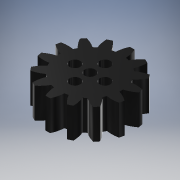
# Autodesk Inventor part: Spur Gear1
Saved by Autodesk Inventor 2017 SP1 (Build 210196100, 196)
## iProperties
Created: 2019-09-22
Part Number: Spur Gear1
Material: ABS Plastic
Document SubType Name: Modeling
Designer: Zach
Categories: <?xml version="1.0" encoding="UTF-16"?> <MemberInstance><Categories><FamilyTemplate><FamilyTemplateParameter ValueType="xs:double" Id="1" ObjectReferenceKey="da_z" ObjectType="kUserParameterObject"/><FamilyTemplateParameter ValueType="xs:double" Id="2" ObjectReferenceKey="da_b" ObjectType="kUserParameterObject"/><FamilyTemplateParameter ValueType="xs:double" Id="3" ObjectReferenceKey="da_beta" ObjectType="kUserParameterObject"/><FamilyTemplateParameter ValueType="xs:double" Id="4" ObjectReferenceKey="da_da" ObjectType="kUserParameterObject"/><FamilyTemplateParameter ValueType="xs:double" Id="5" ObjectReferenceKey="da_aw" ObjectType="kUserParameterObject"/><FamilyTemplateParameter ValueType="xs:string" Id="6" ObjectReferenceKey="EAIAABAAAACIAQAAAAAAAIAAAAAAAAAA" ObjectType="83910656" SubObjectId="SurfaceGeometry"/></FamilyTemplate><ParamToTemplateMap><ParamToTemplate CategoryParameter="//CategoryParameter[@InternalName='046C89C9-8512-4d59-83FE-43B91F4F132A']" TemplateParameter="1"/><ParamToTemplate CategoryParameter="//CategoryParameter[@InternalName='2552DF32-E462-4b46-AEBF-C6C7768E72AC']" TemplateParameter="2"/><ParamToTemplate CategoryParameter="//CategoryParameter[@InternalName='C9EE641D-15FC-4fae-A226-E94C4372FDD7']" TemplateParameter="3"/><ParamToTemplate><ParamToTemplate CategoryParameter="//CategoryParameter[@InternalName='00B6519A-459B-49c7-AD84-2E56D39A5744']" ConstantValue="0.000000"/></ParamToTemplate><ParamToTemplate><ParamToTemplate CategoryParameter="//CategoryParameter[@InternalName='04B31F0E-C7A6-4894-AA32-9629BEFACF47']" ConstantValue="1.000000"/></ParamToTemplate><ParamToTemplate><ParamToTemplate CategoryParameter="//CategoryParameter[@InternalName='43CBEC2E-7847-49e7-A936-2F7889FCB2D9']" ConstantValue="0.250000"/></ParamToTemplate><ParamToTemplate><ParamToTemplate CategoryParameter="//CategoryParameter[@InternalName='B1EFC894-105D-4ebd-86BF-FA20ED196853']" ConstantValue="0.350000"/></ParamToTemplate><ParamToTemplate><ParamToTemplate CategoryParameter="//CategoryParameter[@InternalName='51175063-3D10-4879-93E8-6246FE8B403D']" ConstantValue="2060000000.000000"/></ParamToTemplate><ParamToTemplate><ParamToTemplate CategoryParameter="//CategoryParameter[@InternalName='A3A52E27-4454-46a9-B0BD-C932399B70AF']" ConstantValue="0.300000"/></ParamToTemplate><ParamToTemplate><ParamToTemplate CategoryParameter="//CategoryParameter[@InternalName='91B76062-C214-41d9-B1B9-14D2AB99603D']" ConstantValue="0.180000"/></ParamToTemplate><ParamToTemplate><ParamToTemplate CategoryParameter="//CategoryParameter[@InternalName='374E806E-8B8A-4dda-A9AA-1039D6500AD2']" ConstantValue="5.555556"/></ParamToTemplate><ParamToTemplate><ParamToTemplate CategoryParameter="//CategoryParameter[@InternalName='2D373A89-B862-43d6-8D0B-0CBF12AB9F6C']" ConstantValue="0.392699"/></ParamToTemplate><ParamToTemplate CategoryParameter="//CategoryParameter[@InternalName='37777632-D6A2-4fac-9D53-DB8ACD95C989']" TemplateParameter="4"/><ParamToTemplate CategoryParameter="//CategoryParameter[@InternalName='FD1017F1-B727-4f7e-9707-0F86F1FF9423']" TemplateParameter="5"/><ParamToTemplate><ParamToTemplate CategoryParameter="//CategoryParameter[@InternalName='9E1B4470-B2D3-4ff1-B813-535BB4CDF51A']" ConstantValue="3520000.000000"/></ParamToTemplate><ParamToTemplate><ParamToTemplate CategoryParameter="//CategoryParameter[@InternalName='F8452263-BFF6-458c-9FB1-07C4B99E95CD']" ConstantValue="11400000.000000"/></ParamToTemplate><ParamToTemplate><ParamToTemplate CategoryParameter="//CategoryParameter[@InternalName='3E3BB259-FD49-497f-8171-6EBC954A3479']" ConstantValue="2.000000"/></ParamToTemplate><ParamToTemplate CategoryParameter="//CategoryParameter[@InternalName='27C3BAF2-7550-4e4b-AE2C-0DB134B7D9B7']" TemplateParameter="6"/></ParamToTemplateMap><Category DisplayName="Gear" InternalName="DC85795E-93AB-48d5-8EEE-5A27447B64BD" Mnemonic="Gear"><CategoryParameter DisplayName="z" InternalName="046C89C9-8512-4d59-83FE-43B91F4F132A" Mnemonic="z"/><CategoryParameter DisplayName="b" InternalName="2552DF32-E462-4b46-AEBF-C6C7768E72AC" Mnemonic="b"/><CategoryParameter DisplayName="||b|" InternalName="C9EE641D-15FC-4fae-A226-E94C4372FDD7" Mnemonic="beta"/><CategoryParameter DisplayName="x" InternalName="00B6519A-459B-49c7-AD84-2E56D39A5744" Mnemonic="x"/><CategoryParameter DisplayName="a*" InternalName="04B31F0E-C7A6-4894-AA32-9629BEFACF47" Mnemonic="a"/><CategoryParameter DisplayName="c*" InternalName="43CBEC2E-7847-49e7-A936-2F7889FCB2D9" Mnemonic="c"/><CategoryParameter DisplayName="r|.f|*" InternalName="B1EFC894-105D-4ebd-86BF-FA20ED196853" Mnemonic="rf"/><CategoryParameter DisplayName="E" InternalName="51175063-3D10-4879-93E8-6246FE8B403D" Mnemonic="E"/><CategoryParameter DisplayName="||m|" InternalName="A3A52E27-4454-46a9-B0BD-C932399B70AF" Mnemonic="mi"/><Category DisplayName="SpurGear" InternalName="26C5A22E-A91E-4dfd-A3B3-23CCAFAE1764" Mnemonic="SpurGear"><CategoryParameter DisplayName="m" InternalName="91B76062-C214-41d9-B1B9-14D2AB99603D" Mnemonic="m"/><CategoryParameter DisplayName="P" InternalName="374E806E-8B8A-4dda-A9AA-1039D6500AD2" Mnemonic="PP"/><CategoryParameter DisplayName="||a|" InternalName="2D373A89-B862-43d6-8D0B-0CBF12AB9F6C" Mnemonic="alpha"/><CategoryParameter DisplayName="d|.a|" InternalName="37777632-D6A2-4fac-9D53-DB8ACD95C989" Mnemonic="da"/><CategoryParameter DisplayName="a|.w|" InternalName="FD1017F1-B727-4f7e-9707-0F86F1FF9423" Mnemonic="aw"/><CategoryParameter DisplayName="||s||.Flim|" InternalName="9E1B4470-B2D3-4ff1-B813-535BB4CDF51A" Mnemonic="sFlim"/><CategoryParameter DisplayName="||s||.Hlim|" InternalName="F8452263-BFF6-458c-9FB1-07C4B99E95CD" Mnemonic="sHlim"/><CategoryParameter DisplayName="type" InternalName="3E3BB259-FD49-497f-8171-6EBC954A3479" Mnemonic="type"/><CategoryParameter DisplayName="PitchDiameter" InternalName="27C3BAF2-7550-4e4b-AE2C-0DB134B7D9B7" Mnemonic="IDS_PITCHDIAM"/></Category></Category></Categories></MemberInstance>
Density: 1.06 g/cm^3
Appearance: Smooth - Black
CustomPartVersion: 1
Author: Zach
Autodesk Inventor part; units mm, degrees
ref_plane "YZ Plane" through (0, 0, 0) normal (1, 0, 0) x (0, 1, 0)
ref_plane "XZ Plane" through (0, 0, 0) normal (0, 1, 0) x (-1, 0, 0)
ref_plane "XY Plane" through (0, 0, 0) normal (0, 0, 1) x (1, 0, 0)
sketch "Sketch1" plane through (0, 0, 0) normal (0, 0, 1) x (1, 0, 0)
  circle A0 centre (0, 0) radius 14
  dimension "d0" = 28
  constraints: 1 centre point
  measures "d0" diameter of A0
extrude "Extrusion1" add sketch "Sketch1" along normal blind 10
ref_plane "Work Plane2" through (0, 0, 5) normal (0, 0, 1) x (1, 0, 0)
sketch "Sketch2" plane through (0, 0, 0) normal (0, 0, -1) x (-1, 0, 0)
  circle A0 centre (0, 0) radius 14 projected
  circle A1 centre (0, 0) radius 12.7647
  dimension "d3" = 25.5294
  constraints: 1 centre point, 1 coincident
  measures "d3" diameter of A1
surface extrude "Pitch Diameter" sketch "Sketch2" against normal through all shown no curves A1
ref_plane "Work Plane8" through (0, 0, 0) normal (0.9749279, 0.2225209, 0) x (0, 0, 1)
ref_plane "Work Plane9" through (0, 0, 0) normal (1, 0, 0) x (0, 1, 0)
spur gear teeth "Spur Gear" teeth 14 pitch diameter 25.2 tip diameter 28 root diameter 20.7 face width 10 start plane through (0, 0, 0) normal (0, 0, -1) x (-1, 0, 0)
sketch "Sketch4" plane through (0, 0, 10) normal (0, 0, 1) x (1, 0, 0)
  circle A0 centre (0, 0) radius 16
  circle A1 centre (12, 0) radius 2.5
  circle A2 centre (12, 0) radius 4.5
  circle A3 centre (0, 0) radius 7.5
  dimension "d49" = 32
  dimension "d50" = 5
  dimension "d51" = 12
  dimension "d52" = 9
  constraints: 4 centre point, 3 coincident, 1 horizontal alignment, 1 tangent
  measures "d49" diameter of A0
  measures "d50" diameter of A1
  measures "d51" distance of point (0, 0) A1.centre
  measures "d52" diameter of A2
extrude "Extrusion2" [suppressed]
sketch "Sketch5" plane through (0, 0, 16) normal (0, 0, 1) x (1, 0, 0)
  circle A0 centre (0, 0) radius 16
  circle A1 centre (12, 0) radius 2.5
  circle A2 centre (0, 12) radius 2.5
  circle A3 centre (-12, 0) radius 2.5
  circle A4 centre (0, -12) radius 2.5
  dimension "d55" = 32
  dimension "d56" = 5
  dimension "d57" = 12
  dimension "d60" = 360
  constraints: 5 centre point, 1 coincident, 1 horizontal alignment, 9 other
  measures "d55" diameter of A0
  measures "d56" diameter of A1
  measures "d57" distance of A1.centre point (0, 0)
extrude "Extrusion3" [suppressed]
sketch "Sketch6" plane through (0, 0, 18) normal (0, 0, 1) x (1, 0, 0)
  circle A0 centre (0, -12) radius 2.5 projected
  line L0 (2.5, -12) -> (2.5, -16)
  line L1 (2.5, -16) -> (-2.5, -16)
  line L2 (-2.5, -16) -> (-2.5, -12)
  circle A1 centre (0, 0) radius 16 construction
  arc A2 (2.5, -12) -> (-2.5, -12) centre (0, -12) ccw
  line L3 (12, 2.5) -> (16, 2.5)
  line L4 (16, 2.5) -> (16, -2.5)
  line L5 (16, -2.5) -> (12, -2.5)
  arc A3 (12, 2.5) -> (12, -2.5) centre (12, 0) ccw
  line L6 (-2.5, 12) -> (-2.5, 16)
  line L7 (-2.5, 16) -> (2.5, 16)
  line L8 (2.5, 16) -> (2.5, 12)
  arc A4 (-2.5, 12) -> (2.5, 12) centre (0, 12) ccw
  line L9 (-12, -2.5) -> (-16, -2.5)
  line L10 (-16, -2.5) -> (-16, 2.5)
  line L11 (-16, 2.5) -> (-12, 2.5)
  arc A5 (-12, -2.5) -> (-12, 2.5) centre (-12, 0) ccw
  point P0 (12, 0)
  point P1 (0, 12)
  point P2 (-12, 0)
  dimension "d66" = 360
  constraints: 24 end point, 10 point on circle, 5 tangent, 4 centre point, 1 horizontal alignment, 1 perpendicular, 1 vertical, 41 other
extrude "Extrusion4" [suppressed]
sketch "Sketch7" plane through (0, 0, 13) normal (0, 0, -1) x (-1, 0, 0)
  arc A0 (6.7721, 12.2531) -> (5.3576, 12.9343) centre (0, 0) ccw projected
  arc A1 (-2.5, 12) -> (2.5, 12) centre (0, 12) ccw projected
  arc A2 (-12, -2.5) -> (-12, 2.5) centre (-12, 0) ccw projected
  arc A3 (2.5, -12) -> (-2.5, -12) centre (0, -12) ccw projected
  arc A4 (12, 2.5) -> (12, -2.5) centre (12, 0) ccw projected
  circle A5 centre (0, 12) radius 4.5
  circle A6 centre (-12, 0) radius 4.5
  circle A7 centre (0, -12) radius 4.5
  circle A8 centre (12, 0) radius 4.5
  arc A9 (0.785, 13.978) -> (-0.785, 13.978) centre (0, 0) ccw projected
  arc A10 (5.9892, 8.4411) -> (6.7721, 12.2531) centre (-4.1276, 12.505) ccw projected
  arc A11 (5.3576, 12.9343) -> (2.8652, 9.9455) centre (12.3503, 4.5696) ccw projected
  arc A12 (2.8652, 9.9455) -> (1.7337, 10.2038) centre (0, 0) ccw projected
  arc A13 (1.7337, 10.2038) -> (0.785, 13.978) centre (-9.1446, 9.4757) ccw projected
  arc A14 (-0.785, 13.978) -> (-1.7337, 10.2038) centre (9.1446, 9.4757) ccw projected
  arc A15 (-1.7337, 10.2038) -> (-2.8652, 9.9455) centre (0, 0) ccw projected
  arc A16 (-2.8652, 9.9455) -> (-5.3576, 12.9343) centre (-12.3503, 4.5696) ccw projected
  arc A17 (-5.3576, 12.9343) -> (-6.7721, 12.2531) centre (0, 0) ccw projected
  arc A18 (-6.7721, 12.2531) -> (-5.9892, 8.4411) centre (4.1276, 12.505) ccw projected
  arc A19 (-5.9892, 8.4411) -> (-6.8967, 7.7174) centre (0, 0) ccw projected
  arc A20 (-6.8967, 7.7174) -> (-10.439, 9.3289) centre (-13.11, -1.2415) ccw projected
  arc A21 (-10.439, 9.3289) -> (-11.4179, 8.1014) centre (0, 0) ccw projected
  arc A22 (-11.4179, 8.1014) -> (-9.0586, 5.0065) centre (-1.7068, 13.0575) ccw projected
  arc A23 (-9.0586, 5.0065) -> (-9.5622, 3.9608) centre (0, 0) ccw projected
  arc A24 (-9.5622, 3.9608) -> (-13.4528, 3.8757) centre (-11.273, -6.8068) ccw projected
  arc A25 (-13.4528, 3.8757) -> (-13.8022, 2.3451) centre (0, 0) ccw projected
  arc A26 (-13.8022, 2.3451) -> (-10.3337, 0.5803) centre (-7.2032, 11.0239) ccw projected
  arc A27 (-10.3337, 0.5803) -> (-10.3337, -0.5803) centre (0, 0) ccw projected
  arc A28 (-10.3337, -0.5803) -> (-13.8022, -2.3451) centre (-7.2032, -11.0239) ccw projected
  arc A29 (-13.8022, -2.3451) -> (-13.4528, -3.8757) centre (0, 0) ccw projected
  arc A30 (-13.4528, -3.8757) -> (-9.5622, -3.9608) centre (-11.273, 6.8068) ccw projected
  arc A31 (-9.5622, -3.9608) -> (-9.0586, -5.0065) centre (0, 0) ccw projected
  arc A32 (-9.0586, -5.0065) -> (-11.4179, -8.1014) centre (-1.7068, -13.0575) ccw projected
  arc A33 (-11.4179, -8.1014) -> (-10.439, -9.3289) centre (0, 0) ccw projected
  arc A34 (-10.439, -9.3289) -> (-6.8967, -7.7174) centre (-13.11, 1.2415) ccw projected
  arc A35 (-6.8967, -7.7174) -> (-5.9892, -8.4411) centre (0, 0) ccw projected
  arc A36 (-5.9892, -8.4411) -> (-6.7721, -12.2531) centre (4.1276, -12.505) ccw projected
  arc A37 (-6.7721, -12.2531) -> (-5.3576, -12.9343) centre (0, 0) ccw projected
  arc A38 (-5.3576, -12.9343) -> (-2.8652, -9.9455) centre (-12.3503, -4.5696) ccw projected
  arc A39 (-2.8652, -9.9455) -> (-1.7337, -10.2038) centre (0, 0) ccw projected
  arc A40 (-1.7337, -10.2038) -> (-0.785, -13.978) centre (9.1446, -9.4757) ccw projected
  arc A41 (-0.785, -13.978) -> (0.785, -13.978) centre (0, 0) ccw projected
  arc A42 (0.785, -13.978) -> (1.7337, -10.2038) centre (-9.1446, -9.4757) ccw projected
  arc A43 (1.7337, -10.2038) -> (2.8652, -9.9455) centre (0, 0) ccw projected
  arc A44 (2.8652, -9.9455) -> (5.3576, -12.9343) centre (12.3503, -4.5696) ccw projected
  arc A45 (5.3576, -12.9343) -> (6.7721, -12.2531) centre (0, 0) ccw projected
  arc A46 (6.7721, -12.2531) -> (5.9892, -8.4411) centre (-4.1276, -12.505) ccw projected
  arc A47 (5.9892, -8.4411) -> (6.8967, -7.7174) centre (0, 0) ccw projected
  arc A48 (6.8967, -7.7174) -> (10.439, -9.3289) centre (13.11, 1.2415) ccw projected
  arc A49 (10.439, -9.3289) -> (11.4179, -8.1014) centre (0, 0) ccw projected
  arc A50 (11.4179, -8.1014) -> (9.0586, -5.0065) centre (1.7068, -13.0575) ccw projected
  arc A51 (9.0586, -5.0065) -> (9.5622, -3.9608) centre (0, 0) ccw projected
  arc A52 (9.5622, -3.9608) -> (13.4528, -3.8757) centre (11.273, 6.8068) ccw projected
  arc A53 (13.4528, -3.8757) -> (13.8022, -2.3451) centre (0, 0) ccw projected
  arc A54 (13.8022, -2.3451) -> (10.3337, -0.5803) centre (7.2032, -11.0239) ccw projected
  arc A55 (10.3337, -0.5803) -> (10.3337, 0.5803) centre (0, 0) ccw projected
  arc A56 (10.3337, 0.5803) -> (13.8022, 2.3451) centre (7.2032, 11.0239) ccw projected
  arc A57 (13.8022, 2.3451) -> (13.4528, 3.8757) centre (0, 0) ccw projected
  arc A58 (13.4528, 3.8757) -> (9.5622, 3.9608) centre (11.273, -6.8068) ccw projected
  arc A59 (9.5622, 3.9608) -> (9.0586, 5.0065) centre (0, 0) ccw projected
  arc A60 (9.0586, 5.0065) -> (11.4179, 8.1014) centre (1.7068, 13.0575) ccw projected
  arc A61 (11.4179, 8.1014) -> (10.439, 9.3289) centre (0, 0) ccw projected
  arc A62 (10.439, 9.3289) -> (6.8967, 7.7174) centre (13.11, -1.2415) ccw projected
  arc A63 (6.8967, 7.7174) -> (5.9892, 8.4411) centre (0, 0) ccw projected
  dimension "d76" = 9
  dimension "d77" = 9
  dimension "d78" = 9
  dimension "d79" = 9
  constraints: 4 centre point, 4 coincident
  measures "d76" diameter of A5
  measures "d77" diameter of A6
  measures "d78" diameter of A7
  measures "d79" diameter of A8
extrude "Extrusion6" [suppressed]
sketch "Sketch8" plane through (0, 0, 13) normal (0, 0, -1) x (-1, 0, 0)
  arc A0 (-2.5, 12) -> (2.5, 12) centre (0, 12) ccw projected
  circle A1 centre (0, 12) radius 4.5
  circle A2 centre (-12, 0) radius 4.5
  circle A3 centre (0, -12) radius 4.5
  circle A4 centre (12, 0) radius 4.5
  point P0 (0, 0)
  dimension "d82" = 9
  dimension "d85" = 360
  constraints: 4 centre point, 1 coincident, 9 other
  measures "d82" diameter of A1
extrude "Extrusion7" [suppressed]
sketch "Sketch18" plane through (0, 0, 10) normal (0, 0, 1) x (1, 0, 0)
  circle A0 centre (5, 0) radius 1.1
  circle A1 centre (0, 5) radius 1.1
  circle A2 centre (-5, 0) radius 1.1
  circle A3 centre (0, -5) radius 1.1
  circle A4 centre (5.6569, 5.6569) radius 1.1
  line L0 (0, 0) -> (5.6569, 5.6569) construction
  line L1 (0, 0) -> (5, 0) construction
  circle A5 centre (-5.6569, 5.6569) radius 1.1
  circle A6 centre (-5.6569, -5.6569) radius 1.1
  circle A7 centre (5.6569, -5.6569) radius 1.1
  circle A8 centre (0, 0) radius 1.1
  arc A9 (0.785, 13.978) -> (-0.785, 13.978) centre (0, 0) ccw projected
  arc A10 (-6.7721, 12.2531) -> (-5.9892, 8.4411) centre (4.1276, 12.505) ccw projected
  arc A11 (-5.3576, 12.9343) -> (-6.7721, 12.2531) centre (0, 0) ccw projected
  arc A12 (-2.8652, 9.9455) -> (-5.3576, 12.9343) centre (-12.3503, 4.5696) ccw projected
  arc A13 (-1.7337, 10.2038) -> (-2.8652, 9.9455) centre (0, 0) ccw projected
  arc A14 (-0.785, 13.978) -> (-1.7337, 10.2038) centre (9.1446, 9.4757) ccw projected
  arc A15 (1.7337, 10.2038) -> (0.785, 13.978) centre (-9.1446, 9.4757) ccw projected
  arc A16 (2.8652, 9.9455) -> (1.7337, 10.2038) centre (0, 0) ccw projected
  arc A17 (5.3576, 12.9343) -> (2.8652, 9.9455) centre (12.3503, 4.5696) ccw projected
  arc A18 (6.7721, 12.2531) -> (5.3576, 12.9343) centre (0, 0) ccw projected
  arc A19 (5.9892, 8.4411) -> (6.7721, 12.2531) centre (-4.1276, 12.505) ccw projected
  arc A20 (6.8967, 7.7174) -> (5.9892, 8.4411) centre (0, 0) ccw projected
  arc A21 (10.439, 9.3289) -> (6.8967, 7.7174) centre (13.11, -1.2415) ccw projected
  arc A22 (11.4179, 8.1014) -> (10.439, 9.3289) centre (0, 0) ccw projected
  arc A23 (9.0586, 5.0065) -> (11.4179, 8.1014) centre (1.7068, 13.0575) ccw projected
  arc A24 (9.5622, 3.9608) -> (9.0586, 5.0065) centre (0, 0) ccw projected
  arc A25 (13.4528, 3.8757) -> (9.5622, 3.9608) centre (11.273, -6.8068) ccw projected
  arc A26 (13.8022, 2.3451) -> (13.4528, 3.8757) centre (0, 0) ccw projected
  arc A27 (10.3337, 0.5803) -> (13.8022, 2.3451) centre (7.2032, 11.0239) ccw projected
  arc A28 (10.3337, -0.5803) -> (10.3337, 0.5803) centre (0, 0) ccw projected
  arc A29 (13.8022, -2.3451) -> (10.3337, -0.5803) centre (7.2032, -11.0239) ccw projected
  arc A30 (13.4528, -3.8757) -> (13.8022, -2.3451) centre (0, 0) ccw projected
  arc A31 (9.5622, -3.9608) -> (13.4528, -3.8757) centre (11.273, 6.8068) ccw projected
  arc A32 (9.0586, -5.0065) -> (9.5622, -3.9608) centre (0, 0) ccw projected
  arc A33 (11.4179, -8.1014) -> (9.0586, -5.0065) centre (1.7068, -13.0575) ccw projected
  arc A34 (10.439, -9.3289) -> (11.4179, -8.1014) centre (0, 0) ccw projected
  arc A35 (6.8967, -7.7174) -> (10.439, -9.3289) centre (13.11, 1.2415) ccw projected
  arc A36 (5.9892, -8.4411) -> (6.8967, -7.7174) centre (0, 0) ccw projected
  arc A37 (6.7721, -12.2531) -> (5.9892, -8.4411) centre (-4.1276, -12.505) ccw projected
  arc A38 (5.3576, -12.9343) -> (6.7721, -12.2531) centre (0, 0) ccw projected
  arc A39 (2.8652, -9.9455) -> (5.3576, -12.9343) centre (12.3503, -4.5696) ccw projected
  arc A40 (1.7337, -10.2038) -> (2.8652, -9.9455) centre (0, 0) ccw projected
  arc A41 (0.785, -13.978) -> (1.7337, -10.2038) centre (-9.1446, -9.4757) ccw projected
  arc A42 (-0.785, -13.978) -> (0.785, -13.978) centre (0, 0) ccw projected
  arc A43 (-1.7337, -10.2038) -> (-0.785, -13.978) centre (9.1446, -9.4757) ccw projected
  arc A44 (-2.8652, -9.9455) -> (-1.7337, -10.2038) centre (0, 0) ccw projected
  arc A45 (-5.3576, -12.9343) -> (-2.8652, -9.9455) centre (-12.3503, -4.5696) ccw projected
  arc A46 (-6.7721, -12.2531) -> (-5.3576, -12.9343) centre (0, 0) ccw projected
  arc A47 (-5.9892, -8.4411) -> (-6.7721, -12.2531) centre (4.1276, -12.505) ccw projected
  arc A48 (-6.8967, -7.7174) -> (-5.9892, -8.4411) centre (0, 0) ccw projected
  arc A49 (-10.439, -9.3289) -> (-6.8967, -7.7174) centre (-13.11, 1.2415) ccw projected
  arc A50 (-11.4179, -8.1014) -> (-10.439, -9.3289) centre (0, 0) ccw projected
  arc A51 (-9.0586, -5.0065) -> (-11.4179, -8.1014) centre (-1.7068, -13.0575) ccw projected
  arc A52 (-9.5622, -3.9608) -> (-9.0586, -5.0065) centre (0, 0) ccw projected
  arc A53 (-13.4528, -3.8757) -> (-9.5622, -3.9608) centre (-11.273, 6.8068) ccw projected
  arc A54 (-13.8022, -2.3451) -> (-13.4528, -3.8757) centre (0, 0) ccw projected
  arc A55 (-10.3337, -0.5803) -> (-13.8022, -2.3451) centre (-7.2032, -11.0239) ccw projected
  arc A56 (-10.3337, 0.5803) -> (-10.3337, -0.5803) centre (0, 0) ccw projected
  arc A57 (-13.8022, 2.3451) -> (-10.3337, 0.5803) centre (-7.2032, 11.0239) ccw projected
  arc A58 (-13.4528, 3.8757) -> (-13.8022, 2.3451) centre (0, 0) ccw projected
  arc A59 (-9.5622, 3.9608) -> (-13.4528, 3.8757) centre (-11.273, -6.8068) ccw projected
  arc A60 (-9.0586, 5.0065) -> (-9.5622, 3.9608) centre (0, 0) ccw projected
  arc A61 (-11.4179, 8.1014) -> (-9.0586, 5.0065) centre (-1.7068, 13.0575) ccw projected
  arc A62 (-10.439, 9.3289) -> (-11.4179, 8.1014) centre (0, 0) ccw projected
  arc A63 (-6.8967, 7.7174) -> (-10.439, 9.3289) centre (-13.11, -1.2415) ccw projected
  arc A64 (-5.9892, 8.4411) -> (-6.8967, 7.7174) centre (0, 0) ccw projected
  dimension "d113" = 2.2
  dimension "d114" = 5
  dimension "d115" = 360
  dimension "d116" = 2.2
  dimension "d117" = 45
  dimension "d118" = 8
  dimension "d119" = 360
  dimension "d120" = 2.2
  constraints: 9 centre point, 4 end point, 3 coincident, 1 horizontal, 1 horizontal alignment, 18 other
  measures "d113" diameter of A0
  measures "d114" distance of L0.start L1.end
  measures "d116" diameter of A4
  measures "d117" angle of L1 L0
  measures "d118" distance of L0.start L0.end
  measures "d120" diameter of A8
extrude "Extrusion13" cut sketch "Sketch18" against normal through all contours A0 | A1 | A2 | A3 | A4 | A5 | A6 | A7 | A8
sketch "Sketch19" plane through (0, 0, 10) normal (0, 0, 1) x (1, 0, 0)
  circle A0 centre (5, 0) radius 1
  circle A1 centre (5, 0) radius 1.75
  circle A2 centre (0, 0) radius 1
  circle A3 centre (0, 0) radius 1.75
  circle A4 centre (5.6569, 5.6569) radius 1
  circle A5 centre (5.6569, 5.6569) radius 1.75
  circle A6 centre (-5.6569, 5.6569) radius 1.75
  circle A7 centre (-5.6569, -5.6569) radius 1.75
  circle A8 centre (5.6569, -5.6569) radius 1.75
  circle A9 centre (0, 5) radius 1.75
  circle A10 centre (-5, 0) radius 1.75
  circle A11 centre (0, -5) radius 1.75
  dimension "d123" = 3.5
  dimension "d124" = 3.5
  dimension "d125" = 3.5
  dimension "d128" = 360
  dimension "d132" = 360
  constraints: 12 centre point, 3 coincident, 18 other
  measures "d123" diameter of A1
  measures "d124" diameter of A3
  measures "d125" diameter of A5
extrude "Extrusion14" cut sketch "Sketch19" against normal blind 3 contours A0 | A1 | A2 | A3 | A4 | A5 | A6 | A7 | A8 | A9 | A10 | A11
sketch "Sketch21" plane through (0, 0, 10) normal (0, 0, 1) x (1, 0, 0)
  circle A0 centre (-5.6569, -5.6569) radius 1.75 projected
  circle A1 centre (-5.6569, 5.6569) radius 1.75 projected
  circle A2 centre (5.6569, 5.6569) radius 1.75 projected
  circle A3 centre (5.6569, -5.6569) radius 1.75 projected
  point P0 (0, 0)
extrude "Extrusion15" add sketch "Sketch21" against normal up to surface (10 mm away) from surface at 0
equation "\"d0\" = da_da"
equation "\"d1\" = da_b"
equation "\"d3\" = da_dw"
equation "\"d16\" = da_aw"
equation "\"d43\" = da_aw"
equation "\"d46\" = da_aw"
equation "\"da_da\" = 28"
equation "\"da_b\" = 10"
equation "\"da_dw\" = 25.529412"
equation "\"da_aw\" = 31"
body "Solid1"
body "Srf1"
